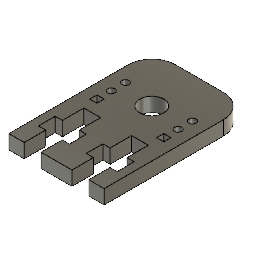
stand_L v10 (Autodesk Fusion 360 design; units mm, degrees)
Autodesk Fusion 360 part; units mm, degrees
note: some values were not read from the file. Set by a fixed rule: which sketch regions a step uses.
sketch "Sketch1" plane through (0, 0, 0) normal (0, 0, 1) x (1, 0, 0)
  line L0 (0, 0) -> (40, 0)
  line L1 (40, 0) -> (40, 60)
  line L2 (40, 60) -> (0, 60)
  line L3 (0, 60) -> (0, 0)
  line L4 (20, 60) -> (20, 27.089)
  circle A0 centre (20, 40) radius 5
  line L5 (6.5, 0) -> (13.5, 0)
  line L6 (13.5, 0) -> (13.5, 25)
  line L7 (13.5, 25) -> (6.5, 25)
  line L8 (6.5, 25) -> (6.5, 0)
  line L9 (26.5, 0) -> (33.5, 0)
  line L10 (33.5, 0) -> (33.5, 25)
  line L11 (33.5, 25) -> (26.5, 25)
  line L12 (26.5, 25) -> (26.5, 0)
  line L13 (10, 25) -> (30, 25)
  line L14 (20, 25) -> (20, 0)
  line L15 (0, 16) -> (40, 16)
  line L16 (3.5, 16) -> (16.5, 16)
  line L17 (16.5, 16) -> (16.5, 9)
  line L18 (16.5, 9) -> (3.5, 9)
  line L19 (3.5, 9) -> (3.5, 16)
  line L20 (3.5, 12.5) -> (6.5, 12.5)
  line L21 (10, 9) -> (10, 0)
  line L22 (23.5, 16) -> (23.5, 9)
  line L23 (23.5, 9) -> (36.5, 9)
  line L24 (36.5, 9) -> (36.5, 16)
  dimension "d1" = 40
  dimension "d2" = 60
  dimension "d3" = 10
  dimension "d4" = 40
  dimension "d5" = 7
  dimension "d6" = 7
  dimension "d7" = 25
  dimension "d8" = 25
  dimension "d9" = 20
  dimension "d10" = 90
  dimension "d11" = 90
  dimension "d12" = 13
  dimension "d13" = 90
  dimension "d14" = 7
  constraint horizontal L0
  constraint vertical L1
  constraint horizontal L2
  constraint vertical L3
  constraint coincident L0.start L3.end
  constraint midpoint L2 L4.start
  constraint perpendicular L2 L4
  constraint coincident L4 A0.centre
  constraint horizontal L5
  constraint vertical L6
  constraint horizontal L7
  constraint vertical L8
  constraint coincident L0 L5.start
  constraint horizontal L9
  constraint vertical L10
  constraint horizontal L11
  constraint vertical L12
  constraint coincident L0 L9.start
  constraint midpoint L7 L13.start
  constraint midpoint L11 L13.end
  constraint midpoint L13 L14.start
  constraint midpoint L0 L14.end
  constraint coincident L3 L15.start
  constraint coincident L1 L15.end
  constraint perpendicular L1 L15
  constraint horizontal L16
  constraint vertical L17
  constraint horizontal L18
  constraint vertical L19
  constraint coincident L15 L16.start
  constraint midpoint L19 L20.start
  constraint midpoint L8 L20.end
  constraint midpoint L18 L21.start
  constraint midpoint L5 L21.end
  constraint symmetric L14 L16.start L24.end
  constraint symmetric L14 L16.end L22.start
  constraint symmetric L14 L17.end L22.end
  constraint symmetric L14 L18.end L23.end
  measures "d1" distance of L0.start L0.end
  measures "d2" distance of L0.end L1.end
  measures "d3" diameter of A0
  measures "d4" distance of L0 A0.centre
  measures "d5" distance of L6.end L7.end
  measures "d6" distance of L10.end L11.end
  measures "d7" distance of L5.start L7.end
  measures "d8" distance of L9.end L10.end
  measures "d9" distance of L13.start L13.end
  measures "d10" angle of L0 L14
  measures "d11" angle of L8 L20
  measures "d12" distance of L17.end L18.end
  measures "d13" angle of L18 L21 L9.start
  measures "d14" distance of L16.end L17.end
extrude "Extrude1" add sketch "Sketch1" along normal blind 6 contours L0 L3 L8 L15 L18 L19 | L1 L2 L3 L7 L8 L10 L11 L13 L15 L16 | L0 L6 L14 L15 L17 L18 | L0 L12 L14 L15 L22 L23 | L6 L13 L14 L15 L16 | L12 L13 L14 L15 | L0 L1 L10 L15 L23 L24
sketch "Sketch2" plane through (0, 0, 6) normal (0, 0, 1) x (-1, 0, 0)
  circle A0 centre (-20, -40) radius 5
  line L0 (-33.5, 0) -> (-40, 0)
  line L1 (-40, 0) -> (-40, -60)
  line L2 (-40, -60) -> (0, -60)
  line L3 (0, -60) -> (0, 0)
  line L4 (0, 0) -> (-6.5, 0)
  line L5 (-6.5, 0) -> (-6.5, -9)
  line L6 (-6.5, -9) -> (-3.5, -9)
  line L7 (-3.5, -9) -> (-3.5, -16)
  line L8 (-3.5, -16) -> (-6.5, -16)
  line L9 (-6.5, -16) -> (-6.5, -25)
  line L10 (-6.5, -25) -> (-13.5, -25)
  line L11 (-13.5, -25) -> (-13.5, -16)
  line L12 (-13.5, -16) -> (-16.5, -16)
  line L13 (-16.5, -16) -> (-16.5, -9)
  line L14 (-16.5, -9) -> (-13.5, -9)
  line L15 (-13.5, -9) -> (-13.5, 0)
  line L16 (-13.5, 0) -> (-26.5, 0)
  line L17 (-26.5, 0) -> (-26.5, -9)
  line L18 (-26.5, -9) -> (-23.5, -9)
  line L19 (-23.5, -9) -> (-23.5, -16)
  line L20 (-23.5, -16) -> (-26.5, -16)
  line L21 (-26.5, -16) -> (-26.5, -25)
  line L22 (-26.5, -25) -> (-33.5, -25)
  line L23 (-33.5, -25) -> (-33.5, -16)
  line L24 (-33.5, -16) -> (-36.5, -16)
  line L25 (-36.5, -16) -> (-36.5, -9)
  line L26 (-36.5, -9) -> (-33.5, -9)
  line L27 (-33.5, -9) -> (-33.5, 0)
  line L28 (0, -40) -> (-40, -40)
  line L29 (-6, -45) -> (-6, -35)
  circle A1 centre (-6, -43) radius 1.5
  circle A2 centre (-6, -37) radius 1.5
  line L30 (-6, -43) -> (-6, -37)
  line L31 (-6, -40) -> (0, -40)
  line L32 (-20, -40) -> (-20, -45)
  circle A3 centre (-34, -43) radius 1.5
  circle A4 centre (-34, -37) radius 1.5
  dimension "d17" = 6
  dimension "d18" = 3
  dimension "d19" = 3
  dimension "d20" = 6
  dimension "d21" = 90
  constraint coincident L3 L28.start
  constraint coincident L1 L28.end
  constraint perpendicular L1 L28
  constraint perpendicular L28 L29
  constraint coincident L29 A1.centre
  constraint coincident L29 A2.centre
  constraint coincident A1.centre L30.start
  constraint coincident A2.centre L30.end
  constraint midpoint L30 L31.start
  constraint coincident A0.centre L32.start
  constraint coincident A0 L32.end
  constraint vertical L32
  constraint coincident L28 A0.centre
  constraint symmetric A1 L32 A3
  constraint symmetric A2 L32 A4
  measures "d17" distance of L3 L29
  measures "d18" diameter of A1
  measures "d19" diameter of A2
  measures "d20" distance of A1.centre A2.centre
  measures "d21" angle of L3 L31
extrude "Extrude2" cut sketch "Sketch2" against normal blind 5 contours L29 A1 L30 | L29 A1 L30 | L29 A2 L30 | L29 A2 L30 | A3 | A4
sketch "Sketch3" plane through (0, 0, 6) normal (0, 0, 1) x (-1, 0, 0)
  circle A0 centre (-6, -37) radius 1.5
  circle A1 centre (-34, -43) radius 1.5
  circle A2 centre (-6, -43) radius 1.5
  circle A3 centre (-34, -37) radius 1.5
  circle A4 centre (-20, -40) radius 5
  line L0 (-33.5, 0) -> (-40, 0)
  line L1 (-40, 0) -> (-40, -60)
  line L2 (-40, -60) -> (0, -60)
  line L3 (0, -60) -> (0, 0)
  line L4 (0, 0) -> (-6.5, 0)
  line L5 (-6.5, 0) -> (-6.5, -9)
  line L6 (-6.5, -9) -> (-3.5, -9)
  line L7 (-3.5, -9) -> (-3.5, -16)
  line L8 (-3.5, -16) -> (-6.5, -16)
  line L9 (-6.5, -16) -> (-6.5, -25)
  line L10 (-6.5, -25) -> (-13.5, -25)
  line L11 (-13.5, -25) -> (-13.5, -16)
  line L12 (-13.5, -16) -> (-16.5, -16)
  line L13 (-16.5, -16) -> (-16.5, -9)
  line L14 (-16.5, -9) -> (-13.5, -9)
  line L15 (-13.5, -9) -> (-13.5, 0)
  line L16 (-13.5, 0) -> (-26.5, 0)
  line L17 (-26.5, 0) -> (-26.5, -9)
  line L18 (-26.5, -9) -> (-23.5, -9)
  line L19 (-23.5, -9) -> (-23.5, -16)
  line L20 (-23.5, -16) -> (-26.5, -16)
  line L21 (-26.5, -16) -> (-26.5, -25)
  line L22 (-26.5, -25) -> (-33.5, -25)
  line L23 (-33.5, -25) -> (-33.5, -16)
  line L24 (-33.5, -16) -> (-36.5, -16)
  line L25 (-36.5, -16) -> (-36.5, -9)
  line L26 (-36.5, -9) -> (-33.5, -9)
  line L27 (-33.5, -9) -> (-33.5, 0)
  line L28 (0, -31) -> (-40, -31)
  line L29 (-4.5, -32.5) -> (-7.5, -32.5)
  line L30 (-7.5, -32.5) -> (-7.5, -29.5)
  line L31 (-7.5, -29.5) -> (-4.5, -29.5)
  line L32 (-4.5, -29.5) -> (-4.5, -32.5)
  line L33 (-6, -37) -> (0, -37)
  line L34 (-6, -37) -> (-6, -32.5)
  line L35 (-4.5, -31) -> (0, -31)
  line L36 (-20, -40) -> (-20, -43)
  line L37 (-35.5, -32.5) -> (-32.5, -32.5)
  line L38 (-32.5, -32.5) -> (-32.5, -29.5)
  line L39 (-35.5, -29.5) -> (-35.5, -32.5)
  line L40 (-32.5, -29.5) -> (-35.5, -29.5)
  dimension "d24" = 3
  dimension "d25" = 3
  dimension "d26" = 90
  dimension "d27" = 6
  dimension "d28" = 90
  constraint coincident L3 L28.start
  constraint coincident L1 L28.end
  constraint perpendicular L1 L28
  constraint horizontal L29
  constraint vertical L30
  constraint horizontal L31
  constraint vertical L32
  constraint coincident A0.centre L33.start
  constraint coincident L3 L33.end
  constraint perpendicular L3 L33
  constraint midpoint L29 L34.end
  constraint midpoint L32 L35.start
  constraint coincident A4.centre L36.start
  constraint vertical L36
  constraint symmetric L29.start L36 L37.start
  constraint symmetric L29.end L36 L37.end
  constraint symmetric L30.end L36 L38.end
  constraint symmetric L31.end L36 L39.start
  measures "d24" distance of L29.end L30.end
  measures "d25" distance of L30.end L31.end
  measures "d26" angle of L29 L34
  measures "d27" distance of L28 L33
  measures "d28" angle of L32 L35
extrude "Extrude3" cut sketch "Sketch3" against normal blind 5 contours L28 L29 L30 L32 | L28 L30 L31 L32 | L28 L37 L38 L39 | L28 L38 L39 L40
fillet "Fillet1" radius 10 1 edges at (0, 60, 3)
fillet "Fillet2" radius 10 1 edges at (40, 60, 3)
extrude "Extrude4" cut 6 faces at (6.8158, 43.2169, 1) (6.1827, 37.4654, 1) (6.5, 30.5, 1) (33.5, 30.5, 1) (33.9601, 37.4654, 1) (33.2997, 43.1474, 1) along direction (0, 0, -1) blind 5
